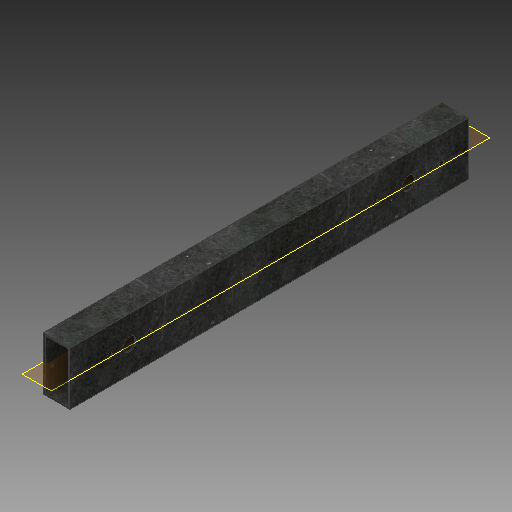
# Autodesk Inventor part: Steel 4130 1x2in. Tubing, t=.065in.,L=15in.
Saved by Autodesk Inventor 2019 (Build 230136000, 136)
## iProperties
Created: 2018-10-28
Part Number: Steel 4130 1x2in. Tubing, t=.065in.,L=15in.
Material: Steel
Document SubType Name: Modeling
Designer: Alex Barnett
Density: 7.85 g/cm^3
Appearance: Plate
Mass: 711.257 g
Surface Area: 1107.15 cm^2
Volume: 90.6059 cm^3
Author: Alex Barnett
Autodesk Inventor part; units mm, degrees
ref_plane "YZ Plane" through (0, 0, 0) normal (1, 0, 0) x (0, 1, 0)
ref_plane "XY Plane" through (0, 0, 0) normal (0, 0, 1) x (1, 0, 0)
sketch "Sketch1" plane through (0, 0, 0) normal (0, 0, 1) x (1, 0, 0)
  line L0 (-12.7, -25.4) -> (12.7, -25.4)
  line L1 (12.7, -25.4) -> (12.7, 25.4)
  line L2 (12.7, 25.4) -> (-12.7, 25.4)
  line L3 (-12.7, 25.4) -> (-12.7, -25.4)
  line L4 (-12.7, -25.4) -> (12.7, 25.4) construction
  line L5 (12.7, -25.4) -> (-12.7, 25.4) construction
  line L6 (-11.049, -23.749) -> (11.049, -23.749)
  line L7 (11.049, -23.749) -> (11.049, 23.749)
  line L8 (11.049, 23.749) -> (-11.049, 23.749)
  line L9 (-11.049, 23.749) -> (-11.049, -23.749)
  line L10 (-11.049, -23.749) -> (11.049, 23.749) construction
  line L11 (11.049, -23.749) -> (-11.049, 23.749) construction
  point P0 (0, 0)
  dimension "d0" = 25.4
  dimension "d1" = 50.8
  dimension "d4" = 22.098
  dimension "d5" = 47.498
  constraints: 24 end point, 4 midpoint, 4 parallel, 2 horizontal, 2 perpendicular
  measures "d0" distance of L2.end L1.end
  measures "d1" distance of L1.end L0.end
  measures "d4" distance of L8.end L7.end
  measures "d5" distance of L7.end L6.end
extrude "Extrusion2" add sketch "Sketch1" along normal mid plane 381
sketch "Sketch3" plane through (12.7, -25.4, 190.5) normal (1, 0, 0) x (0, 0, -1)
  line L0 (381, 50.8) -> (0, 50.8) projected
  line L1 (0, 0) -> (0, 50.8) projected
  line L2 (381, 0) -> (0, 0) projected
  line L3 (381, 50.8) -> (381, 0) projected
  circle A0 centre (57.15, 25.4) radius 6.35
  point P0 (190.5, 25.4)
  dimension "d22" = 12.7
  dimension "d23" = 57.15
  dimension "d24" = 25.4
  constraints: 1 centre point
  measures "d22" diameter of A0
  measures "d23" distance from line of L1 A0.centre
  measures "d24" distance from line of L0 A0.centre
hole "Hole2" at (12.7, 0, 133.35) direction (-1, 0, 0) diameter 12.7 end through all
sketch "Sketch4" plane through (12.7, -25.4, 190.5) normal (1, 0, 0) x (0, 0, -1)
  circle A0 centre (57.15, 25.4) radius 6.35 projected
  line L0 (381, 50.8) -> (0, 50.8) projected
  line L1 (0, 0) -> (0, 50.8) projected
  line L2 (381, 0) -> (0, 0) projected
  line L3 (381, 50.8) -> (381, 0) projected
  point P0 (190.5, 25.4)
  point P1 (323.85, 25.4)
  dimension "d32" = 57.15
  dimension "d33" = 25.4
  measures "d32" distance from line of L3 point (323.85, 25.4)
  measures "d33" distance from line of L0 point (323.85, 25.4)
hole "Hole3" at (12.7, 0, -133.35) direction (-1, 0, 0) diameter 12.7 end through all
sketch "Sketch5" plane through (12.7, -25.4, 190.5) normal (1, 0, 0) x (0, 0, -1)
  circle A0 centre (323.85, 25.4) radius 6.35 projected
  circle A1 centre (57.15, 25.4) radius 6.35 projected
  line L0 (381, 50.8) -> (0, 50.8) projected
  line L1 (0, 0) -> (0, 50.8) projected
  line L2 (381, 0) -> (0, 0) projected
  line L3 (381, 50.8) -> (381, 0) projected
  point P0 (190.5, 25.4)
  point P1 (355.6, 25.4)
  point P2 (292.1, 25.4)
  dimension "d41" = 63.5
  dimension "d42" = 31.75
  measures "d41" distance of point (292.1, 25.4) point (355.6, 25.4)
  measures "d42" distance of A0.centre point (355.6, 25.4)
hole "Hole4" at (12.7, 0, -101.6) at (12.7, 0, -165.1) direction (-1, 0, 0) diameter 5.08 end through all
sketch "Sketch6" plane through (12.7, -25.4, 190.5) normal (1, 0, 0) x (0, 0, -1)
  circle A0 centre (292.1, 25.4) radius 2.54 projected
  circle A1 centre (355.6, 25.4) radius 2.54 projected
  circle A2 centre (323.85, 25.4) radius 6.35 projected
  circle A3 centre (57.15, 25.4) radius 6.35 projected
  line L0 (381, 50.8) -> (0, 50.8) projected
  line L1 (0, 0) -> (0, 50.8) projected
  line L2 (381, 0) -> (0, 0) projected
  line L3 (381, 50.8) -> (381, 0) projected
  circle A4 centre (38.1, 25.4) radius 2.54
  line L4 (57.15, 31.75) -> (57.15, 19.05) construction
  circle A5 centre (76.2, 25.4) radius 2.54
  point P0 (190.5, 25.4)
  dimension "d53" = 5.08
  dimension "d54" = 19.05
  constraints: 2 centre point, 2 end point, 2 point on circle, 1 symmetric about line, 1 vertical, 1 other
  measures "d53" diameter of A4
  measures "d54" distance of A3.centre A4.centre
hole "Hole5" at (12.7, 0, 152.4) at (12.7, 0, 114.3) direction (-1, 0, 0) diameter 5.08 end through all
body "Solid2"
